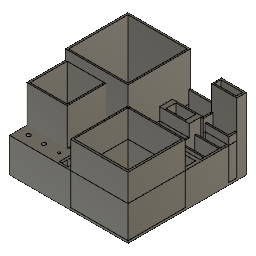
收纳1 (Autodesk Fusion 360 design; units mm, degrees)
part number: 2026-02-27-19-53-02-708
Autodesk Fusion 360 part; units mm, degrees
note: some values were not read from the file. Set by a fixed rule: which sketch regions a step uses.
sketch "草图1" plane through (0, 0, 0) normal (0, 0, 1) x (1, 0, 0)
  line L0 (-120, 120) -> (120, 120)
  line L1 (120, 120) -> (120, -120)
  line L2 (120, -120) -> (-120, -120)
  line L3 (-120, -120) -> (-120, 120)
  line L4 (-120, 120) -> (120, -120) construction
  line L5 (120, 120) -> (-120, -120) construction
  line L6 (-116, -116) -> (-116, 116)
  line L7 (-116, 116) -> (116, 116)
  line L8 (116, 116) -> (116, -116)
  line L9 (116, -116) -> (-116, -116)
  line L10 (-116, 116) -> (4, 116)
  line L11 (4, 116) -> (4, -4)
  line L12 (4, -4) -> (-116, -4)
  line L13 (-116, -4) -> (-116, 116)
  line L14 (7, 116) -> (7, -7)
  line L15 (7, -7) -> (-116, -7)
  line L16 (-91.3834, 29.143) -> (-25.513, 29.143) construction
  line L17 (-25.513, 29.143) -> (-25.513, 88.3753) construction
  line L18 (-25.513, 88.3753) -> (-91.3834, 88.3753) construction
  line L19 (-91.3834, 88.3753) -> (-91.3834, 29.143) construction
  line L20 (7, 80) -> (72, 80)
  line L21 (72, 80) -> (72, 116)
  line L22 (7, 83) -> (69, 83)
  line L23 (69, 83) -> (69, 116)
  line L24 (25.1429, 88.9882) -> (53.1683, 88.9882) construction
  line L25 (53.1683, 88.9882) -> (53.1683, 99.6185) construction
  line L26 (53.1683, 99.6185) -> (25.1429, 99.6185) construction
  line L27 (25.1429, 99.6185) -> (25.1429, 88.9882) construction
  line L28 (67, 80) -> (67, 57)
  line L29 (67, 57) -> (7, 57)
  line L30 (17, 80) -> (57, 80)
  line L31 (57, 80) -> (57, 60)
  line L32 (57, 60) -> (17, 60)
  line L33 (17, 60) -> (17, 80)
  line L34 (26, 65.6005) -> (48.0911, 65.6005) construction
  line L35 (48.0911, 65.6005) -> (48.0911, 73) construction
  line L36 (48.0911, 73) -> (26, 73) construction
  line L37 (26, 73) -> (26, 65.6005) construction
  line L38 (-116, -7) -> (-41, -7)
  line L39 (-41, -7) -> (-41, -82)
  line L40 (-41, -82) -> (-116, -82)
  line L41 (-116, -82) -> (-116, -7)
  line L42 (-38, -7) -> (-38, -85)
  line L43 (-38, -85) -> (-116, -85)
  line L44 (-99.1433, -54.3081) -> (-63.0106, -54.3081) construction
  line L45 (-63.0106, -54.3081) -> (-63.0106, -32.999) construction
  line L46 (-63.0106, -32.999) -> (-99.1433, -32.999) construction
  line L47 (-99.1433, -32.999) -> (-99.1433, -54.3081) construction
  line L48 (7, 57) -> (67, 57)
  line L49 (67, 57) -> (67, 37)
  line L50 (67, 37) -> (7, 37)
  line L51 (7, 37) -> (7, 57)
  line L52 (64, 57) -> (64, 40)
  line L53 (64, 40) -> (7, 40)
  line L54 (25.5114, 42.6447) -> (56.3611, 42.6447) construction
  line L55 (56.3611, 42.6447) -> (56.3611, 51.3132) construction
  line L56 (56.3611, 51.3132) -> (25.5114, 51.3132) construction
  line L57 (25.5114, 51.3132) -> (25.5114, 42.6447) construction
  line L58 (72, 103) -> (116, 103)
  line L59 (72, 87) -> (116, 87)
  line L60 (72, 100) -> (116, 100)
  line L61 (72, 84) -> (116, 84)
  line L62 (67, 71) -> (116, 71)
  line L63 (67, 40) -> (116, 40)
  line L64 (67, 68) -> (116, 68)
  line L65 (67, 37) -> (116, 37)
  line L66 (76.846, 102.1326) -> (102.0197, 102.0197) construction
  line L67 (102.0197, 102.0197) -> (102.0756, 114.498) construction
  line L68 (102.0756, 114.498) -> (76.902, 114.6109) construction
  line L69 (76.902, 114.6109) -> (76.846, 102.1326) construction
  line L70 (84.3585, 90.542) -> (111.7961, 90.6188) construction
  line L71 (111.7961, 90.6188) -> (111.7764, 97.6581) construction
  line L72 (111.7764, 97.6581) -> (84.3388, 97.5814) construction
  line L73 (84.3388, 97.5814) -> (84.3585, 90.542) construction
  line L74 (94.1738, 75) -> (110, 75) construction
  line L75 (110, 75) -> (110, 79.4268) construction
  line L76 (110, 79.4268) -> (94.1738, 79.4268) construction
  line L77 (94.1738, 79.4268) -> (94.1738, 75) construction
  line L78 (80, 47.31) -> (108.2637, 47.31) construction
  line L79 (108.2637, 47.31) -> (108.2637, 60) construction
  line L80 (108.2637, 60) -> (80, 60) construction
  line L81 (80, 60) -> (80, 47.31) construction
  line L82 (-85, -85) -> (-85, -116)
  line L83 (-54, -85) -> (-54, -116)
  line L84 (-38, -85) -> (-5, -85)
  line L85 (-5, -85) -> (-5, -116)
  line L86 (-23, -85) -> (-23, -116)
  line L87 (-116, -85) -> (-85, -116) construction
  line L88 (-54, -85) -> (-85, -116) construction
  line L89 (-85, -85) -> (-54, -116) construction
  line L90 (-54, -85) -> (-23, -116) construction
  line L91 (-23, -116) -> (-5, -85) construction
  line L92 (-23, -85) -> (-5, -116) construction
  line L93 (-23, -85) -> (-54, -116) construction
  circle A0 centre (-100.5, -100.5) radius 3.65
  circle A1 centre (-69.5, -100.5) radius 3.65
  circle A2 centre (-38.5, -100.5) radius 2.25
  circle A3 centre (-14, -100.5) radius 2.5
  line L94 (72, 6) -> (7, 6)
  line L95 (72, 12) -> (72, 6)
  line L96 (26.8319, 6.972) -> (48.9756, 6.972) construction
  line L97 (48.9756, 6.972) -> (48.9756, 11.0156) construction
  line L98 (48.9756, 11.0156) -> (26.8319, 11.0156) construction
  line L99 (26.8319, 11.0156) -> (26.8319, 6.972) construction
  line L100 (40.1808, 17.1326) -> (43.385, 17.1326) construction
  line L101 (43.385, 17.1326) -> (43.385, 35.2897) construction
  line L102 (43.385, 35.2897) -> (40.1808, 35.2897) construction
  line L103 (40.1808, 35.2897) -> (40.1808, 17.1326) construction
  line L104 (18.6537, 18.964) -> (25.5317, 18.964) construction
  line L105 (25.5317, 18.964) -> (25.5317, 32.3581) construction
  line L106 (25.5317, 32.3581) -> (18.6537, 32.3581) construction
  line L107 (18.6537, 32.3581) -> (18.6537, 18.964) construction
  line L108 (35, 37) -> (35, 12)
  line L109 (35, 12) -> (7, 12)
  line L110 (32, 15) -> (7, 15)
  line L111 (32, 37) -> (32, 15)
  line L112 (35, 15) -> (67, 15)
  line L113 (67, 15) -> (67, 37)
  line L114 (35, 12) -> (70, 12)
  line L115 (70, 12) -> (70, 37)
  line L116 (70, 30) -> (116, 30)
  line L117 (70, 27) -> (116, 27)
  line L118 (79.0707, 32.0224) -> (93.9955, 32.0224) construction
  line L119 (93.9955, 32.0224) -> (93.9955, 35.3609) construction
  line L120 (93.9955, 35.3609) -> (79.0707, 35.3609) construction
  line L121 (79.0707, 35.3609) -> (79.0707, 32.0224) construction
  line L122 (7, -7) -> (116, -7)
  line L123 (116, -7) -> (116, -116)
  line L124 (116, -116) -> (7, -116)
  line L125 (7, -116) -> (7, -7)
  line L126 (7, 116) -> (7, 120)
  line L127 (-116, -7) -> (-121.1752, -7)
  line L128 (72, 116) -> (72, 120)
  line L129 (116, 100) -> (120, 100)
  line L130 (116, 84) -> (120, 84)
  line L131 (69, 116) -> (69, 120)
  line L132 (72, 100) -> (69, 100)
  line L133 (72, 84) -> (69, 84)
  line L134 (-38, -7) -> (-38, -4)
  line L135 (-116, -85) -> (-120, -85)
  line L136 (-116, -4) -> (-120, -4)
  line L137 (86.5, 23) -> (86.5, -4)
  line L138 (74.7536, 23) -> (74.7536, 3)
  line L139 (84, -4.0797) -> (84, 23)
  line L140 (113.5, -4) -> (113.5, 23)
  line L141 (86.5, -4) -> (113.5, -4)
  line L142 (113.5, 23) -> (86.5, 23)
  line L143 (84, 23) -> (74.7536, 23)
  line L144 (7, -4.0797) -> (84, -4.0797)
  line L145 (74.7536, 3) -> (7, 3)
  line L146 (7, 3) -> (7, -4.0797)
  line L147 (4.0918, -82) -> (-38, -82)
  line L148 (-38, -7) -> (4, -7)
  line L149 (-38, -27) -> (-38, -7)
  line L150 (-38, -50) -> (-38, -30)
  line L151 (-38, -30) -> (4, -30)
  line L152 (-38, -82) -> (-38, -54.2912)
  line L153 (4, -27) -> (-38, -27)
  line L154 (4, -50) -> (-38, -50)
  line L155 (-38, -54.2912) -> (4.0918, -54.2912)
  line L156 (4.0918, -54.2912) -> (4.0918, -82)
  line L157 (4, -30) -> (4, -50)
  line L158 (4, -7) -> (4, -27)
  line L159 (72, 12) -> (70, 12)
  line L160 (84, -4.0797) -> (116, -4.0797)
  line L161 (4, -7) -> (4, -120)
  line L162 (116, -4.0797) -> (120, -4.0797)
  circle A4 centre (-38.5, -100.5) radius 5.25
  circle A5 centre (-69.5, -100.5) radius 6.65
  circle A6 centre (-100.5, -100.5) radius 6.65
  circle A7 centre (-14, -100.5) radius 5.5
  point P0 (66.165, 12.6159)
  point P1 (18.6537, 18.964)
  point P2 (18.6537, 32.3581)
  point P3 (25.5317, 18.964)
  point P4 (25.5317, 32.3581)
  dimension "d22" = 240
  dimension "d23" = 240
  dimension "d24" = 4
  dimension "d25" = 120
  dimension "d26" = 120
  dimension "d28" = 10
  dimension "d45" = 65
  dimension "d46" = 36
  dimension "d47" = -3
  dimension "d48" = 5
  dimension "d50" = 44
  dimension "d51" = 60
  dimension "d52" = 23
  dimension "d54" = 40
  dimension "d55" = 20
  dimension "d56" = 10
  dimension "d57" = 5
  dimension "d60" = 75
  dimension "d61" = 75
  dimension "d62" = -3
  dimension "d63" = 5
  dimension "d65" = 60
  dimension "d66" = 20
  dimension "d67" = 3
  dimension "d68" = 5
  dimension "d70" = 13
  dimension "d76" = 3
  dimension "d77" = 3
  dimension "d80" = 13
  dimension "d81" = 3
  dimension "d82" = 3
  dimension "d84" = 5
  dimension "d86" = 5
  dimension "d88" = 5
  dimension "d90" = 5
  dimension "d92" = 13
  dimension "d93" = 60
  dimension "d100" = 31
  dimension "d101" = 31
  dimension "d102" = 31
  dimension "d103" = 31
  dimension "d104" = 18
  dimension "d105" = 7.3
  dimension "d106" = 7.3
  dimension "d107" = 4.5
  dimension "d108" = 5
  dimension "d119" = 5
  dimension "d122" = 5
  dimension "d125" = 5
  dimension "d127" = -3
  dimension "d128" = 25
  dimension "d129" = 22
  dimension "d131" = 32
  dimension "d132" = 22
  dimension "d133" = 3
  dimension "d134" = 7
  dimension "d135" = 3
  dimension "d136" = 5
  dimension "d138" = 109
  dimension "d139" = 109
  dimension "d144" = 65
  dimension "d145" = 6
  dimension "d255" = 27
  dimension "d256" = 27
  dimension "d257" = 42
  dimension "d258" = 20
  dimension "d259" = 42
  dimension "d260" = 20
  dimension "d261" = 3
  dimension "d263" = 2.5
  dimension "d264" = 2.5
  dimension "d265" = 4
  dimension "d275" = 3
  dimension "d276" = 3
  dimension "d277" = 3
  dimension "d280" = 3
  constraint horizontal L0
  constraint perpendicular L0 L1
  constraint parallel L0 L2
  constraint parallel L1 L3
  constraint coincident L4 origin
  constraint coincident L5 origin
  constraint horizontal L10
  constraint vertical L11
  constraint horizontal L12
  constraint vertical L13
  constraint coincident L7 L14.start
  constraint coincident L6 L15.end
  constraint coincident L14 L20.start
  constraint perpendicular L14 L20
  constraint coincident L7 L21.end
  constraint perpendicular L7 L21
  constraint coincident L20 L28.start
  constraint perpendicular L20 L28
  constraint coincident L14 L29.end
  constraint perpendicular L14 L29
  constraint horizontal L30
  constraint vertical L31
  constraint horizontal L32
  constraint vertical L33
  constraint coincident L20 L30.start
  constraint horizontal L38
  constraint vertical L39
  constraint horizontal L40
  constraint vertical L41
  constraint horizontal L48
  constraint vertical L49
  constraint horizontal L50
  constraint vertical L51
  constraint coincident L21 L58.start
  constraint perpendicular L8 L58
  constraint coincident L8 L58.end
  constraint coincident L28 L62.start
  constraint coincident L8 L62.end
  constraint perpendicular L8 L62
  constraint coincident L49 L63.start
  constraint coincident L8 L63.end
  constraint perpendicular L8 L63
  constraint coincident L5
  constraint coincident L50 L49.end
  constraint coincident L43 L82.start
  constraint coincident L9 L82.end
  constraint perpendicular L9 L82
  constraint coincident L43 L83.start
  constraint coincident L9 L83.end
  constraint perpendicular L9 L83
  constraint perpendicular L42 L84
  constraint coincident L9 L85.end
  constraint perpendicular L9 L85
  constraint coincident L84 L86.start
  constraint coincident L9 L86.end
  constraint perpendicular L9 L86
  constraint perpendicular L5 L87
  constraint midpoint L87 A0.centre
  constraint midpoint L89 A1.centre
  constraint midpoint L93 A2.centre
  constraint midpoint L91 A3.centre
  constraint coincident L50 L111.start
  constraint coincident L14 L110.end
  constraint perpendicular L110 L111
  constraint coincident L108 L112.start
  constraint perpendicular L101 L112
  constraint perpendicular L50 L113
  constraint coincident L115 L116.start
  constraint coincident L8 L116.end
  constraint perpendicular L8 L116
  constraint horizontal L122
  constraint vertical L123
  constraint horizontal L124
  constraint vertical L125
  constraint perpendicular L94 L95
  constraint coincident L0 L126.end
  constraint perpendicular L0 L126
  constraint perpendicular L3 L127
  constraint coincident L0 L128.end
  constraint perpendicular L0 L128
  constraint coincident L1 L129.end
  constraint perpendicular L1 L129
  constraint coincident L1 L130.end
  constraint perpendicular L1 L130
  constraint coincident L0 L131.end
  constraint perpendicular L0 L131
  constraint coincident L23 L132.end
  constraint perpendicular L23 L132
  constraint coincident L23 L133.end
  constraint perpendicular L23 L133
  constraint coincident L12 L134.end
  constraint perpendicular L12 L134
  constraint coincident L3 L135.end
  constraint perpendicular L3 L135
  constraint coincident L3 L136.end
  constraint perpendicular L3 L136
  constraint horizontal L141
  constraint vertical L140
  constraint horizontal L142
  constraint vertical L137
  constraint vertical L146
  constraint perpendicular L144 L146
  constraint perpendicular L139 L144
  constraint perpendicular L139 L143
  constraint perpendicular L138 L143
  constraint horizontal L145
  constraint horizontal L153
  constraint vertical L149
  constraint horizontal L151
  constraint vertical L157
  constraint horizontal L154
  constraint vertical L150
  constraint horizontal L155
  constraint vertical L156
  constraint horizontal L147
  constraint vertical L152
  constraint collinear L149 L150
  constraint collinear L150 L152
  constraint collinear L142 L143
  constraint collinear L14 L146
  constraint coincident L8 L160.end
  constraint perpendicular L8 L160
  constraint coincident L2 L161.end
  constraint perpendicular L2 L161
  constraint coincident L1 L162.end
  constraint perpendicular L1 L162
  measures "d22" distance of L1.end L2.end
  measures "d23" distance of L0.end L1.end
  measures "d25" distance of L6.end L10.end
  measures "d26" distance of L6.end L12.end
  measures "d45" distance of L14 L21
  measures "d46" distance of L7 L20
  measures "d50" distance of L8 L21
  measures "d51" distance of L14 L28
  measures "d52" distance of L20 L29
  measures "d54" distance of L30.start L30.end
  measures "d55" distance of L30.start L32.end
  measures "d56" distance of L14 L33
  measures "d60" distance of L15.end L38.end
  measures "d61" distance of L15.end L40.end
  measures "d65" distance of L29.end L28.end
  measures "d66" distance of L29.end L50.end
  measures "d70" distance of L7 L58
  measures "d80" distance of L61 L62
  measures "d92" distance of L59 L60
  measures "d93" distance of L14 L28
  measures "d100" distance of L9 L43
  measures "d101" distance of L6 L82
  measures "d102" distance of L82 L83
  measures "d103" distance of L83 L86
  measures "d104" distance of L85 L86
  measures "d105" diameter of A0
  measures "d106" diameter of A1
  measures "d107" diameter of A2
  measures "d108" diameter of A3
  measures "d128" distance of L14 L111
  measures "d129" distance of L50 L110
  measures "d131" distance of L112.start L112.end
  measures "d132" distance of L50 L112
  measures "d134" distance of L65 L116
  measures "d138" distance of L9 L122
  measures "d139" distance of L8 L125
  measures "d144" distance of L14 L95
  measures "d145" distance of L94 L114
  measures "d255" distance of L137.end L140.start
  measures "d256" distance of L137.end L137.start
  measures "d257" distance of L42.start L148.end
  measures "d258" distance of L42.start L149.start
  measures "d259" distance of L151.end L150.end
  measures "d260" distance of L150.end L150.start
  measures "d261" distance of L151 L153
  measures "d263" distance of L8 L140
  measures "d264" distance of L137 L139
  measures "d265" distance of L117 L142
sketch "草图2" plane through (0, 0, 0) normal (0, 0, 1) x (1, 0, 0)
  line L0 (-120, 120) -> (120, 120)
  line L1 (120, 120) -> (120, -120)
  line L2 (120, -120) -> (-120, -120)
  line L3 (-120, -120) -> (-120, 120)
  circle A0 centre (-14, -100.5) radius 2.5
  circle A1 centre (-38.5, -100.5) radius 2.25
  circle A2 centre (-69.5, -100.5) radius 3.65
  circle A3 centre (-100.5, -100.5) radius 3.65
  line L4 (3.9913, -3.998) -> (-116.0052, -3.998)
  line L5 (3.9913, 116.0345) -> (3.9913, -3.998)
  line L6 (7.0361, -7.055) -> (116, -7.055)
  line L7 (7.0361, -116.055) -> (7.0361, -7.055)
  line L8 (-116.0087, 116.002) -> (3.9913, 116.0345)
  line L9 (-116.0052, -3.998) -> (-116.0087, 116.002)
  line L10 (116, -7.055) -> (116, -116.055)
  line L11 (116, -116.055) -> (7.0361, -116.055)
  line L12 (-41, -7) -> (-41, -82)
  line L13 (-41, -82) -> (-116, -82)
  line L14 (-116, -116) -> (-116, 116.0345)
  line L15 (-41, -7) -> (-116, -7)
  line L16 (32, 37) -> (32, 15)
  line L17 (32, 15) -> (7, 15)
  line L18 (35, 15) -> (67, 15)
  line L19 (67, 15) -> (67, 37)
  line L20 (35, 37) -> (35, 15)
  line L21 (72, 6) -> (7, 6)
  line L22 (72, 12) -> (72, 6)
  line L23 (35, 12) -> (70, 12)
  line L24 (35, 12) -> (7, 12)
  line L25 (70, 30) -> (116, 30)
  line L26 (70, 30) -> (70, 37)
  line L27 (67, 40) -> (116, 40)
  line L28 (67, 57) -> (67, 40)
  line L29 (67, 68.0345) -> (116, 68.0345)
  line L30 (64, 57) -> (64, 39.9995)
  line L31 (64, 39.9995) -> (7, 39.9995)
  line L32 (57, 80.0345) -> (57, 60.0345)
  line L33 (57, 60.0345) -> (17, 60.0345)
  line L34 (17, 60.0345) -> (17, 80.0345)
  line L35 (7, 83.0345) -> (69, 83.0345)
  line L36 (69, 83.0345) -> (69, 116.005)
  line L37 (17, 80.0345) -> (57, 80.0345)
  line L38 (72, 84.0345) -> (116, 84.0345)
  line L39 (67, 71.0345) -> (116, 71.0345)
  line L40 (72, 87.0345) -> (116, 87.0345)
  line L41 (72, 103.0345) -> (116, 103.0345)
  line L42 (72, 100.0345) -> (116, 100.0345)
  line L43 (3.5986, -3.998) -> (3.9913, -3.998)
  line L44 (7, 12) -> (7, 6)
  line L45 (7, 37) -> (7, 15)
  line L46 (32, 37) -> (7, 37)
  line L47 (67, 37) -> (35, 37)
  line L48 (70, 37) -> (116, 37)
  line L49 (72, 12) -> (70, 12)
  line L50 (67, 68.0345) -> (67, 57)
  line L51 (67, 80.0345) -> (67, 71.0345)
  line L52 (116, 100.0345) -> (116, 87.0345)
  line L53 (116, 116.0403) -> (116, 103.0345)
  line L54 (72, 103.0345) -> (72, 116.0345)
  line L55 (72, 80.0368) -> (72, 84.0345)
  line L56 (72, 87.0345) -> (72, 100.0345)
  line L57 (17, 80.0345) -> (57, 80.0345)
  line L58 (67, 80.0345) -> (72, 80.0368)
  line L59 (-116, 116.0345) -> (3.9913, 116.0345)
  line L60 (7, 116.0345) -> (69, 116.005)
  line L61 (72, 116.0345) -> (116, 116.0403)
  line L62 (7, 116.0345) -> (7, 83.0345)
  line L63 (7, 57) -> (7, 39.9995)
  line L64 (116, 84.0345) -> (116, 71.0345)
  line L65 (116, -7.055) -> (116, -116)
  line L66 (116, 68.0345) -> (116, 40)
  line L67 (116, 37) -> (116, 30)
  line L68 (7, 57) -> (64, 57)
  line L69 (-38, -7) -> (4, -7)
  line L70 (4, -7) -> (4, -27)
  line L71 (4, -27) -> (-38, -27)
  line L72 (-38, -27) -> (-38, -7)
  line L73 (4, -30) -> (4, -50)
  line L74 (-38, -50) -> (-38, -30)
  line L75 (4, -50) -> (-38, -50)
  line L76 (-38, -30) -> (4, -30)
  line L77 (-38, -54.2912) -> (4.0918, -54.2912)
  line L78 (4.0918, -54.2912) -> (4.0918, -82)
  line L79 (4.0918, -82) -> (-38, -82)
  line L80 (-38, -82) -> (-38, -54.2912)
  line L81 (113.5, 23) -> (86.5, 23)
  line L82 (74.7536, 23) -> (74.7536, 3)
  line L83 (113.5, -4) -> (113.5, 23)
  line L84 (84, -4.0797) -> (84, 23)
  line L85 (86.5, -4) -> (113.5, -4)
  line L86 (86.5, 23) -> (86.5, -4)
  line L87 (84, 23) -> (74.7536, 23)
  line L88 (74.7536, 3) -> (7, 3)
  line L89 (7, -4.0797) -> (84, -4.0797)
  line L90 (7, 3) -> (7, -4.0797)
  line L91 (7, 116) -> (7, 83.0345)
  line L92 (7, 57) -> (7, 39.9995)
  line L93 (7, 37) -> (7, 6)
  dimension "d176" = 7.3
  dimension "d177" = 7.3
  dimension "d178" = 4.5
  dimension "d179" = 5
  dimension "d180" = 120
  dimension "d181" = 120
  dimension "d186" = 3
  dimension "d187" = 3
  dimension "d188" = 3
  dimension "d193" = 65
  dimension "d194" = 36
  dimension "d197" = 40
  dimension "d198" = 20
  dimension "d199" = 10
  dimension "d200" = 75
  dimension "d201" = 75
  dimension "d202" = 13
  dimension "d203" = 13
  dimension "d204" = 13
  dimension "d206" = 25
  dimension "d208" = 32
  dimension "d212" = 65
  dimension "d213" = 6
  dimension "d215" = 3
  dimension "d227" = 42
  dimension "d228" = 20
  dimension "d230" = 42
  dimension "d231" = 20
  dimension "d232" = 3.002
  dimension "d233" = 3
  dimension "d236" = 3
  dimension "d266" = 27
  dimension "d267" = 27
  dimension "d268" = 2.5
  constraint horizontal L0
  constraint vertical L1
  constraint horizontal L2
  constraint vertical L3
  constraint vertical L5
  constraint horizontal L4
  constraint horizontal L6
  constraint vertical L7
  constraint coincident L60.start L59
  constraint coincident L15.end L14
  constraint perpendicular L57 L63
  constraint coincident L54.end L59
  constraint perpendicular L55 L59
  constraint coincident L51.start L57
  constraint horizontal L37
  constraint vertical L32
  constraint horizontal L33
  constraint vertical L34
  constraint vertical L12
  constraint horizontal L13
  constraint vertical L28
  constraint coincident L17.end L63
  constraint perpendicular L16 L17
  constraint perpendicular L21 L22
  constraint horizontal L46
  constraint horizontal L47
  constraint coincident L26 L48.start
  constraint perpendicular L50 L57
  constraint perpendicular L51 L57
  constraint perpendicular L41 L53
  constraint perpendicular L54 L59
  constraint collinear L62 L63
  constraint coincident L39 L64.end
  constraint collinear L64 L66
  constraint coincident L25 L67.end
  constraint collinear L65 L67
  constraint coincident L27 L66.end
  constraint collinear L66 L67
  constraint horizontal L68
  constraint horizontal L71
  constraint vertical L72
  constraint horizontal L76
  constraint vertical L73
  constraint horizontal L75
  constraint vertical L74
  constraint horizontal L77
  constraint vertical L78
  constraint horizontal L79
  constraint vertical L80
  constraint collinear L72 L74
  constraint collinear L74 L80
  constraint collinear L13 L79
  constraint horizontal L85
  constraint vertical L83
  constraint horizontal L81
  constraint vertical L86
  constraint perpendicular L84 L89
  constraint perpendicular L84 L87
  constraint perpendicular L82 L87
  constraint horizontal L88
  constraint collinear L81 L87
  constraint collinear L90 L93
  constraint collinear L91 L92
  constraint collinear L92 L93
  measures "d176" diameter of A3
  measures "d177" diameter of A2
  measures "d178" diameter of A1
  measures "d179" diameter of A0
  measures "d180" distance of L5.start L8.start
  measures "d181" distance of L4.end L8.start
  measures "d193" distance of L55 L62
  measures "d194" distance of L57 L59
  measures "d197" distance of L34.end L32.start
  measures "d198" distance of L34.end L33.end
  measures "d199" distance of L34 L63
  measures "d200" distance of L15.end L12.start
  measures "d201" distance of L15.end L13.end
  measures "d202" distance of L41 L59
  measures "d203" distance of L38 L39
  measures "d204" distance of L40 L42
  measures "d206" distance of L16 L63
  measures "d208" distance of L18.start L18.end
  measures "d212" distance of L22 L63
  measures "d213" distance of L21 L23
  measures "d215" distance of L27 L47
  measures "d227" distance of L69.start L69.end
  measures "d228" distance of L69.start L71.end
  measures "d230" distance of L74.end L73.start
  measures "d231" distance of L74.end L74.start
  measures "d232" distance of L4 L69
  measures "d233" distance of L71 L76
  measures "d236" distance of L12 L72
  measures "d266" distance of L83.start L85.start
  measures "d267" distance of L81.end L85.start
  measures "d268" distance of L84 L86
sketch "草图3" plane through (0, 0, 0) normal (0, 0, 1) x (1, 0, 0)
  line L0 (-120, 120) -> (120, 120)
  line L1 (-120, -120) -> (-120, 120)
  line L2 (120, 120) -> (120, -120)
  line L3 (120, -120) -> (-120, -120)
  point P0 (116, 40)
  constraint horizontal L0
  constraint vertical L2
  constraint horizontal L3
  constraint vertical L1
extrude "拉伸2" add sketch "草图3" against normal blind 5 makes body 1
extrude "拉伸3" add sketch "草图2" along normal blind 65 bodies 1
extrude "拉伸4" add sketch "草图1" along normal blind 160 contours L0 L3 L6 L7 L10 L13 L126 L136 | L3 L6 L127 L136 | L7 L11 L12 L14 L15 L51 L134 L146 L148 | L6 L12 L15 L38 L134 bodies 1
extrude "拉伸5" add sketch "草图1" along normal blind 90 contours L0 L7 L126 L131 | L0 L7 L128 L131 | L7 L21 L23 L132 | L14 L20 L21 L22 L23 L30 L133 | L21 L23 L132 L133 | L14 L20 L28 L29 L31 L32 L33 L48 bodies 1
extrude "拉伸6" add sketch "草图1" along normal blind 140 contours L0 L1 L7 L8 L128 L129 | L8 L21 L58 L60 bodies 1
extrude "拉伸7" add sketch "草图1" along normal blind 140 contours L0 L7 L128 L131 | L7 L21 L23 L132 bodies 1
extrude "拉伸8" add sketch "草图1" along normal blind 80 separate body contours L1 L8 L129 L130 | L8 L21 L59 L61 makes body 2
extrude "拉伸9" add sketch "草图1" along normal blind 140 separate body contours L3 L6 L127 L136 | L3 L6 L41 L127 L135 | L6 L12 L15 L38 L134 | L6 L15 L39 L40 L42 L43 L149 L150 L152 makes body 3
extrude "拉伸10" add sketch "草图1" along normal blind 120 separate body contours L1 L2 L8 L9 L123 L124 L161 L162 | L9 L15 L125 L147 L155 L156 L157 L158 L161 | L8 L14 L122 L144 L160 makes body 4
extrude "拉伸11" cut sketch "草图1" along normal blind 70 contours L9 L84 L85 L86 | A7 bodies 1
extrude "拉伸12" add sketch "草图1" along normal blind 40 separate body contours L9 L84 L85 L86 | A7 makes body 5
extrude "拉伸13" cut sketch "草图1" along normal blind 60 contours L6 L9 L43 L82 | L9 L43 L82 L83 | L9 L43 L83 L84 L86 bodies 1
extrude "拉伸14" cut sketch "草图1" along normal blind 30 contours L9 L84 L85 L86 bodies 5
equation "d29 = '胶带160'"
equation "d49 = '大钳95 '"
equation "d58 = '小钳95'"
equation "d64 = '杂物140'"
equation "d69 = '电工钳95 '"
equation "d85 = '卡尺140'"
equation "d87 = '扳手80 '"
equation "d89 = '铲子70'"
equation "d91 = '电子尺60'"
equation "d120 = '剪刀65'"
equation "d123 = '小刀70'"
equation "d126 = '电笔70'"
equation "d137 = '杂物60 '"
